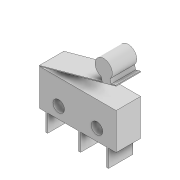
# Autodesk Inventor part: 00_MicroSwitch
Saved by Autodesk Inventor 2022 (Build 260153000, 153)
## iProperties
Created: 2021-09-23
Part Number: 00_MicroSwitch
Material: Generic
Document SubType Name: Modeling
Designer: wanghaoran
Density: 1 g/cm^3
Appearance: Default
Author: wanghaoran
Autodesk Inventor part; units mm, degrees
ref_plane "YZ Plane" through (0, 0, 0) normal (1, 0, 0) x (0, 1, 0)
ref_plane "XZ Plane" through (0, 0, 0) normal (0, 1, 0) x (-1, 0, 0)
ref_plane "XY Plane" through (0, 0, 0) normal (0, 0, 1) x (1, 0, 0)
sketch "Sketch1" plane through (0, 0, 0) normal (0, 0, 1) x (1, 0, 0)
  line L0 (0, 0) -> (20, 0)
  line L1 (20, 0) -> (20, 9.5)
  line L2 (20, 9.5) -> (0, 9.5)
  line L3 (0, 9.5) -> (0, 0)
  circle A0 centre (5, 3) radius 1.5
  circle A1 centre (15, 3) radius 1.5
  dimension "d0" = 20
  dimension "d1" = 9.5
  dimension "d4" = 3
  dimension "d5" = 3
  dimension "d6" = 5
  constraints: 8 end point, 2 centre point, 2 parallel, 1 horizontal, 1 perpendicular
  measures "d0" distance of L2.end L1.end
  measures "d1" distance of L1.end L0.end
  measures "d4" diameter of A0
  measures "d5" diameter of A1
  measures "d6" distance from line of L1 A1.centre
extrude "Extrusion1" add sketch "Sketch1" along normal blind 6.4
sketch "Sketch2" plane through (0, 0, 6.4) normal (0, 0, 1) x (1, 0, 0)
  line L0 (20, 0) -> (20, 9.5) projected
  line L1 (20, 9.5) -> (20, 15)
  line L2 (20, 9.5) -> (0, 9.5) projected
  line L3 (20, 15) -> (0, 9.5)
  line L4 (0, 9.5) -> (-0.053, 9.6928)
  line L5 (20, 15) -> (19.947, 15.1928)
  line L6 (-0.053, 9.6928) -> (19.947, 15.1928)
  circle A0 centre (16.7417, 17.4228) radius 2.25
  line L7 (15.8961, 15.9357) -> (16.3709, 14.2094)
  line L8 (18.2287, 16.5772) -> (18.7035, 14.8509)
  arc A1 (18.2287, 16.5772) -> (15.8961, 15.9357) centre (17.0624, 16.2565) ccw
  point P0 (0, 0)
  point P1 (18.4111, 15.9142)
  point P2 (16.0785, 15.2727)
  dimension "d7" = 5.5
  dimension "d8" = 0.2
  dimension "d9" = 270
  dimension "d10" = 0.2
  dimension "d13" = 4.5
  dimension "d28" = 3
  constraints: 14 end point, 3 perpendicular, 3 point on circle, 2 centre point, 2 point on line, 2 tangent, 1 vertical
  measures "d7" distance of L0.end L1.end
  measures "d8" distance of L2.end L4.end
  measures "d10" distance of L5.start L5.end
  measures "d13" diameter of A0
  measures "d28" distance from line of L6 A0.centre
extrude "Extrusion2" add sketch "Sketch2" against normal blind 6.4 contours L3 L4 L6 L5 | L6 L7 A0 L8 | L8 A1 L7 A0 | A0 L7 A1 L8
sketch "Sketch3" plane through (0, 0, 6.4) normal (0, 0, 1) x (1, 0, 0)
  line L0 (1.6, 0) -> (2.1, 0)
  line L1 (2.1, 0) -> (2.1, -4.6)
  line L2 (2.1, -4.6) -> (1.6, -4.6)
  line L3 (1.6, -4.6) -> (1.6, 0)
  line L4 (0, 0) -> (20, 0) projected
  line L5 (10.7, 0) -> (10.2, 0)
  line L6 (10.2, 0) -> (10.2, -4.6)
  line L7 (10.2, -4.6) -> (10.7, -4.6)
  line L8 (10.7, -4.6) -> (10.7, 0)
  line L9 (18, 0) -> (17.5, 0)
  line L10 (17.5, 0) -> (17.5, -4.6)
  line L11 (17.5, -4.6) -> (18, -4.6)
  line L12 (18, -4.6) -> (18, 0)
  line L13 (0, 9.5) -> (0, 0) projected
  dimension "d16" = 1.6
  dimension "d17" = 0.5
  dimension "d18" = 4.6
  dimension "d20" = 0.5
  dimension "d21" = 8.1
  dimension "d23" = 0.5
  dimension "d24" = 6.8
  dimension "d25" = 4.6
  constraints: 24 end point, 6 parallel, 4 point on line, 3 horizontal, 3 perpendicular
  measures "d16" distance between parallel lines of L13 L3
  measures "d17" distance between parallel lines of L1 L3
  measures "d18" distance of L0.end L1.end
  measures "d20" distance of L6.end L7.end
  measures "d21" distance between parallel lines of L1 L6
  measures "d23" distance of L10.end L11.end
  measures "d24" distance between parallel lines of L10 L8
  measures "d25" distance of L5.end L6.end
extrude "Extrusion3" add sketch "Sketch3" against normal blind 6.4
body "Solid1"
